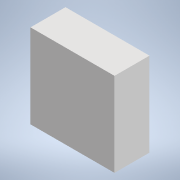
# Autodesk Inventor part: Pieza2
Saved by Autodesk Inventor 2020 (Build 240168000, 168)
## iProperties
Created: 2021-01-20
Part Number: Pieza2
Material: Genérico
Document SubType Name: Modeling
Designer: DanielAlvaradoPelaez
Density: 1 g/cm^3
Appearance: Valor por defecto
Author: DanielAlvaradoPelaez
Autodesk Inventor part; units mm, degrees
ref_plane "YZ Plane" through (0, 0, 0) normal (1, 0, 0) x (0, 1, 0)
ref_plane "XZ Plane" through (0, 0, 0) normal (0, 1, 0) x (-1, 0, 0)
ref_plane "XY Plane" through (0, 0, 0) normal (0, 0, 1) x (1, 0, 0)
sketch "Boceto1" plane through (0, 0, 0) normal (0, 0, 1) x (1, 0, 0)
  line L0 (-12, -12) -> (12, -12)
  line L1 (12, -12) -> (12, 12)
  line L2 (12, 12) -> (-12, 12)
  line L3 (-12, 12) -> (-12, -12)
  line L4 (-12, -12) -> (12, 12) construction
  line L5 (12, -12) -> (-12, 12) construction
  point P0 (0, 0)
  dimension "d0" = 24
  dimension "d1" = 24
  constraints: 12 end point, 2 midpoint, 2 parallel, 1 horizontal, 1 perpendicular
  measures "d0" distance of L2.end L1.end
  measures "d1" distance of L1.end L0.end
extrude "Extrusión1" add sketch "Boceto1" along normal blind 10
